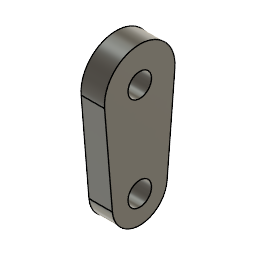
leg joint_12mm (Autodesk Fusion 360 design; units mm, degrees)
part number: 2026-02-05-17-56-03-611
Autodesk Fusion 360 part; units mm, degrees
sketch "Sketch1" plane through (0, 0, 0) normal (1, 0, 0) x (0, 1, 0)
  circle A0 centre (0, 0) radius 1.5
  circle A1 centre (0, -12) radius 1.5
  circle A2 centre (0, 0) radius 4.5
  circle A3 centre (0, -12) radius 3.5
  line L0 (-4.4843, -0.375) -> (-3.4878, -12.2917)
  line L1 (4.4843, -0.375) -> (3.4878, -12.2917)
  dimension "d1" = 3
  dimension "d2" = 3
  dimension "d3" = 12
  dimension "d4" = 7
  dimension "d5" = 9
  constraint coincident A0.centre A2.centre
  constraint concentric A0 A2
  constraint concentric A1 A3
  constraint coincident A2 L0.start
  constraint coincident A3 L0.end
  constraint tangent A2 L0
  constraint tangent A3 L0
  constraint vertical A0.centre A1.centre
  constraint coincident A2 L1.start
  constraint coincident A3 L1.end
  constraint tangent A2 L1
  constraint tangent A3 L1
  measures "d1" diameter of A0
  measures "d2" diameter of A1
  measures "d3" distance of A0.centre A1.centre
  measures "d4" diameter of A3
  measures "d5" diameter of A2
extrude "Extrude1" add sketch "Sketch1" along normal blind 3
